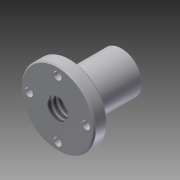
# Autodesk Inventor part: ZACMENut
Saved by Autodesk Inventor 2015 SP1 (Build 190203100, 203)
## iProperties
Category: Hardware
Created: 2014-01-02
Part Number: ZACMENut
Material: ABS Plastic
Document SubType Name: Modeling
Designer: Jack
Density: 1.06 g/cm^3
Appearance: Smooth - White
Mass: 6.03264 g
Surface Area: 32.9386 cm^2
Volume: 5.69117 cm^3
Vendor: MakersToolWorks
Author: Jack
Title: Z Axis Leadscrew Nut
Autodesk Inventor part; units mm, degrees
ref_plane "YZ Plane" through (0, 0, 0) normal (1, 0, 0) x (0, 1, 0)
ref_plane "XZ Plane" through (0, 0, 0) normal (0, 1, 0) x (-1, 0, 0)
ref_plane "XY Plane" through (0, 0, 0) normal (0, 0, 1) x (1, 0, 0)
sketch "Sketch1" plane through (0, 0, 0) normal (0, 1, 0) x (-1, 0, 0)
  circle A0 centre (0, 0) radius 14.25
  dimension "d0" = 28.5
  constraints: 1 centre point, 1 coincident
  measures "d0" diameter of A0
extrude "Extrusion1" add sketch "Sketch1" along normal blind 5
sketch "Sketch2" plane through (0, 5, 0) normal (0, 1, 0) x (1, 0, 0)
  circle A0 centre (0, 0) radius 14.25 projected
  circle A1 centre (0, 0) radius 7.9
  dimension "d3" = 15.8
  constraints: 1 centre point, 1 coincident
  measures "d3" diameter of A1
extrude "Extrusion2" add sketch "Sketch2" along normal blind 20 contours A1
sketch "Sketch3" plane through (0, 25, 0) normal (0, 1, 0) x (1, 0, 0)
  circle A0 centre (0, 0) radius 7.9 projected
  circle A1 centre (0, 0) radius 4
  dimension "d6" = 8
  constraints: 1 centre point, 1 coincident
  measures "d6" diameter of A1
extrude "Extrusion3" cut sketch "Sketch3" against normal blind 25.6 contours A1
chamfer "Chamfer1" distance 0.5 angle 45 1 edges at (-7.9, 25, 0)
chamfer "Chamfer2" distance 0.5 angle 45 3 edges at (-7.9, 5, 0) (14.25, 5, 0) (14.25, 0, 0)
thread "Thread1" size "TR10x2" class "7H" standard "ISO Metric Trapezoidal Threads" full length
sketch "Sketch5" plane through (0, 0, 0) normal (0, -1, 0) x (1, 0, 0)
  circle A0 centre (0, 0) radius 4 projected
  circle A1 centre (0, 0) radius 13.75 projected
  line L0 (0, 0) -> (-13.75, 0) construction
  line L1 (0, 0) -> (13.75, 0) construction
  circle A2 centre (0, 0) radius 13.75 construction
  line L2 (0, 0) -> (0, 13.75) construction
  line L3 (0, 0) -> (0, -13.75) construction
  circle A3 centre (0, 11) radius 1.5
  circle A4 centre (11, 0) radius 1.5
  circle A5 centre (-11, 0) radius 1.5
  circle A6 centre (0, -11) radius 1.5
  dimension "d28" = 11
  dimension "d29" = 3
  dimension "d30" = 11
  dimension "d31" = 11
  dimension "d32" = 11
  constraints: 8 end point, 7 point on circle, 4 centre point, 4 point on line, 3 equal radius, 2 collinear, 1 horizontal, 1 perpendicular
  measures "d28" distance of A0.centre A3.centre
  measures "d29" diameter of A3
  measures "d30" distance of A6.centre A0.centre
  measures "d31" distance of A0.centre A5.centre
  measures "d32" distance of A4.centre A0.centre
extrude "Extrusion5" cut sketch "Sketch5" against normal up to surface (5 mm away) contours A3 | A4 | A5 | A6
body "Solid1"
